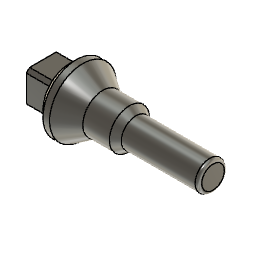
Shaft02 (Autodesk Fusion 360 design; units mm, degrees)
Autodesk Fusion 360 part; units mm, degrees
sketch "Sketch1" plane through (0, 0, 0) normal (0, 1, 0) x (1, 0, 0) in component "Shaft02"
  line L0 (0, 0) -> (0, 40)
  line L1 (0, 40) -> (10, 50)
  line L2 (0, 40) -> (22.4585, 40) construction
  line L3 (10, 50) -> (10, 0)
  line L4 (0, 0) -> (50, 0)
  line L5 (50, 0) -> (50, 30)
  line L6 (10, 50) -> (20, 50)
  line L7 (20, 50) -> (50, 30)
  line L8 (50, 0) -> (90, 0)
  line L9 (90, 0) -> (90, 30)
  line L10 (90, 30) -> (50, 30)
  line L11 (50, 30) -> (50, 0)
  line L12 (90, 0) -> (100, 0)
  line L13 (90, 30) -> (100, 22)
  line L14 (100, 0) -> (216, 0)
  line L15 (216, 0) -> (216, 22)
  line L16 (216, 22) -> (100, 22)
  line L17 (100, 22) -> (100, 0)
  dimension "d2" = 40
  dimension "d3" = 45
  dimension "d5" = 50
  dimension "d6" = 50
  dimension "d7" = 30
  dimension "d8" = 10
  dimension "d10" = 40
  dimension "d11" = 30
  dimension "d13" = 10
  dimension "d15" = 116
  dimension "d16" = 22
  constraint coincident L0.start L4.start
  constraint horizontal L2
  constraint perpendicular L0 L4
  constraint perpendicular L3 L6
  constraint horizontal L8
  constraint vertical L9
  constraint horizontal L10
  constraint vertical L11
  constraint horizontal L12
  constraint horizontal L14
  constraint vertical L15
  constraint horizontal L16
  constraint vertical L17
  measures "d2" distance of L0.start L0.end
  measures "d3" angle of L1 L2
  measures "d5" distance of L1.end L3.end
  measures "d6" distance of L0.start L4.end
  measures "d7" distance of L4.end L5.end
  measures "d8" distance of L1.end L6.end
  measures "d10" distance of L4.end L8.end
  measures "d11" distance of L4.end L5.end
  measures "d13" distance of L8.end L12.end
  measures "d15" distance of L12.end L14.end
  measures "d16" distance of L12.end L13.end
revolve "Revolve1" add sketch "Sketch1" angle 360 about axis through (100, 0, 0) along (1, 0, 0) in component "Shaft02"
sketch "Sketch2" plane through (0, 0, 0) normal (-1, 0, 0) x (0, -1, 0) in component "Shaft02"
  circle A0 centre (0, 0) radius 40
  line L0 (25, -25) -> (-25, -25)
  line L1 (-25, -25) -> (-25, 25)
  line L2 (-25, 25) -> (25, 25)
  line L3 (25, 25) -> (25, -25)
  line L4 (25, -25) -> (-25, 25) construction
  line L5 (-25, -25) -> (25, 25) construction
  dimension "d19" = 50
  dimension "d20" = 50
  constraint horizontal L0
  constraint perpendicular L0 L1
  constraint parallel L0 L2
  constraint parallel L1 L3
  constraint coincident L4 A0.centre
  constraint coincident L5 A0.centre
  constraint coincident A0.centre origin
  measures "d19" distance of L1.end L2.end
  measures "d20" distance of L0.end L1.end
extrude "Extrude1" add sketch "Sketch2" along normal blind 40 contours L0 L1 L2 L3 in component "Shaft02"
chamfer "Chamfer1" distance 5 angle 45 4 edges at (-20, -25, 25) (-20, 25, 25) (-20, -25, -25) (-20, 25, -25) in component "Shaft02"
fillet "Fillet1" radius 5 1 edges at (216, -7.9555, 20.5112) in component "Shaft02"
component "Shaft02" placed x (1, 0, 0) y (0, 1, 0) z (0, 0, 1) at (0, 0, 0)
